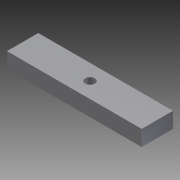
# Autodesk Inventor part: cetakan sepatu 5
Saved by Autodesk Inventor 2012 (Build 160160000, 160)
## iProperties
Created: 2014-01-20
Part Number: cetakan sepatu 5
Material: Default
Document SubType Name: Modeling
Designer: Irwan Haryanto
Density: 1 g/cm^3
Author: Irwan Haryanto
Autodesk Inventor part; units mm, degrees
ref_plane "YZ Plane" through (0, 0, 0) normal (1, 0, 0) x (0, 1, 0)
ref_plane "XZ Plane" through (0, 0, 0) normal (0, 1, 0) x (-1, 0, 0)
ref_plane "XY Plane" through (0, 0, 0) normal (0, 0, 1) x (1, 0, 0)
sketch "Sketch1" plane through (0, 0, 0) normal (0, 0, 1) x (1, 0, 0)
  line L0 (-38.7713, -146.7705) -> (-38.7713, -136.7705)
  line L1 (-38.7713, -136.7705) -> (4.2287, -136.7705)
  line L2 (4.2287, -136.7705) -> (4.2287, -146.7705)
  line L3 (4.2287, -146.7705) -> (-38.7713, -146.7705)
  circle A0 centre (-17.2713, -141.7705) radius 1.5
  line L4 (-38.7713, -146.7705) -> (-38.7713, -136.7705)
  line L5 (-38.7713, -136.7705) -> (4.2287, -136.7705)
  line L6 (4.2287, -136.7705) -> (4.2287, -146.7705)
  line L7 (4.2287, -146.7705) -> (-38.7713, -146.7705)
  circle A1 centre (-17.2713, -141.7705) radius 1.5
  point P0 (0, 0)
  dimension "d0" = 3
  dimension "d1" = 5
  dimension "d2" = 21.5
  dimension "d3" = 3
  dimension "d4" = 5
  dimension "d5" = 21.5
  constraints: 16 end point, 4 perpendicular, 2 centre point, 2 parallel
  measures "d0" diameter of A0
  measures "d1" distance from line of L1 A0.centre
  measures "d2" distance from line of L0 A0.centre
  measures "d3" diameter of A1
  measures "d4" distance from line of L5 A1.centre
  measures "d5" distance from line of L4 A1.centre
extrude "Extrusion1" add sketch "Sketch1" along normal blind 5
body "Solid1"
